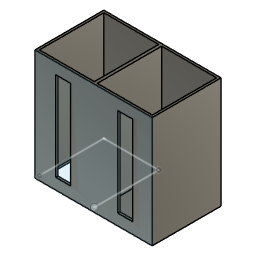
Container (Autodesk Fusion 360 design; units mm, degrees)
Autodesk Fusion 360 part; units mm, degrees
sketch "Szkic1" plane through (0, 0, 0) normal (0, 0, 1) x (1, 0, 0)
  line L0 (0, 0) -> (158.35, 0)
  line L1 (158.35, 0) -> (158.35, 93)
  line L2 (158.35, 93) -> (0, 93)
  line L3 (0, 93) -> (0, 0)
  line L4 (3, 5) -> (3, 3)
  line L5 (3, 3) -> (5, 3)
  line L6 (3, 3) -> (155.35, 3)
  line L7 (155.35, 3) -> (155.35, 90)
  line L8 (155.35, 90) -> (3, 90)
  line L9 (3, 90) -> (3, 3)
  dimension "d1" = 158.35
  dimension "d2" = 93
  dimension "d3" = 152.35
  dimension "d4" = 87
  constraint horizontal L0
  constraint vertical L1
  constraint horizontal L2
  constraint vertical L3
  constraint coincident L0.start L3.end
  constraint horizontal L6
  constraint vertical L7
  constraint horizontal L8
  constraint vertical L9
  measures "d1" distance of L0.start L0.end
  measures "d2" distance of L0.start L2.end
  measures "d3" distance of L4.end L6.end
  measures "d4" distance of L4.end L8.end
extrude "Wyciągnięcie proste1" add sketch "Szkic1" along normal blind 150
sketch "Szkic2" plane through (0, 90, 0) normal (0, -1, 0) x (1, 0, 0)
  line L0 (3, 0) -> (155.35, 0)
  line L1 (155.35, 0) -> (155.35, 150)
  line L2 (155.35, 150) -> (3, 150)
  line L3 (3, 150) -> (3, 0)
  line L4 (79.175, 150) -> (77.175, 150)
  line L5 (77.175, 150) -> (81.175, 150)
  line L6 (81.175, 150) -> (81.175, 0)
  line L7 (81.175, 0) -> (77.175, 0)
  line L8 (77.175, 0) -> (77.175, 150)
  dimension "d7" = 2
  dimension "d8" = 4
  constraint midpoint L2 L4.start
  constraint horizontal L5
  constraint vertical L6
  constraint horizontal L7
  constraint vertical L8
  measures "d7" distance of L4.start L4.end
  measures "d8" distance of L4.end L5.end
extrude "Wyciągnięcie proste2" add sketch "Szkic2" along normal blind 87 contours L0 L2 L4 L5 L6 L7 L8
sketch "Szkic3" plane through (0, 0, 0) normal (0, -1, 0) x (1, 0, 0)
  line L0 (0, 0) -> (158.35, 0)
  line L1 (158.35, 0) -> (158.35, 150)
  line L2 (158.35, 150) -> (0, 150)
  line L3 (0, 150) -> (0, 0)
sketch "Szkic4" plane through (0, 0, 0) normal (0, 0, -1) x (1, 0, 0)
  line L0 (81.175, -3) -> (155.35, -3)
  line L1 (155.35, -3) -> (155.35, -90)
  line L2 (155.35, -90) -> (81.175, -90)
  line L3 (81.175, -90) -> (81.175, -3)
  line L4 (77.175, -3) -> (77.175, -90)
  line L5 (77.175, -90) -> (3, -90)
  line L6 (3, -90) -> (3, -3)
  line L7 (3, -3) -> (77.175, -3)
  line L8 (0, 0) -> (0, -93)
  line L9 (0, -93) -> (158.35, -93)
  line L10 (158.35, -93) -> (158.35, 0)
  line L11 (158.35, 0) -> (0, 0)
  line L12 (0, 0) -> (158.35, 0)
  line L13 (158.35, 0) -> (158.35, -93)
  line L14 (158.35, -93) -> (0, -93)
  line L15 (0, -93) -> (0, 0)
  constraint horizontal L12
  constraint vertical L13
  constraint horizontal L14
  constraint vertical L15
  constraint coincident L9.end L10.start
  constraint coincident L8.start L11.end
extrude "Wyciągnięcie proste3" add sketch "Szkic4" against normal blind 3 contours L0 L1 L2 L3 | L4 L5 L6 L7
sketch "Szkic5" plane through (0, 0, 0) normal (0, -1, 0) x (1, 0, 0)
  line L0 (40, 15) -> (38.0507, 15)
  line L1 (38.0507, 15) -> (28.0507, 15)
  line L2 (28.0507, 15) -> (48.0507, 15)
  line L3 (48.0507, 15) -> (48.0507, 135)
  line L4 (48.0507, 135) -> (28.0507, 135)
  line L5 (28.0507, 135) -> (28.0507, 15)
  line L6 (131.9493, 135) -> (131.9493, 15)
  line L7 (120, 15) -> (121.9493, 15)
  line L8 (111.9493, 135) -> (131.9493, 135)
  line L9 (121.9493, 15) -> (131.9493, 15)
  line L10 (131.9493, 15) -> (111.9493, 15)
  line L11 (111.9493, 15) -> (111.9493, 135)
  dimension "d13" = 10
  dimension "d14" = 20
  dimension "d15" = 120
  constraint horizontal L2
  constraint vertical L3
  constraint horizontal L4
  constraint vertical L5
  measures "d13" distance of L0.end L1.end
  measures "d14" distance of L1.end L2.end
  measures "d15" distance of L1.end L4.end
extrude "Wyciągnięcie proste4" cut sketch "Szkic5" against normal blind 10
sketch "Szkic6" plane through (0, 0, 3) normal (0, 0, 1) x (-1, 0, 0)
  line L0 (-3, -90) -> (-3, -3)
  line L1 (-3, -3) -> (-77.175, -3)
  line L2 (-77.175, -3) -> (-77.175, -90)
  line L3 (-77.175, -90) -> (-3, -90)
  line L4 (-77.175, -3) -> (-77.175, -90)
  line L5 (-77.175, -90) -> (-3, -90)
  line L6 (-3, -90) -> (-3, -3)
  line L7 (-3, -90) -> (-5, -90)
  constraint vertical L4
  constraint horizontal L5
  constraint vertical L6
  constraint coincident L2.end L3.start
  constraint coincident L0.end L1.start
  constraint coincident L5 L7.end
  constraint perpendicular L0 L7
sketch "Szkic7" plane through (0, 0, 3) normal (0, 0, 1) x (-1, 0, 0)
  line L0 (-77.175, -90) -> (-77.175, -3)
  line L1 (-77.175, -3) -> (-77.175, -5)
  line L2 (-75.175, -5) -> (-5, -5)
  line L3 (-5, -5) -> (-5, -88)
  line L4 (-5, -88) -> (-75.175, -88)
  line L5 (-75.175, -88) -> (-75.175, -5)
  point P0 (-5, -90)
  point P1 (-77.175, -3)
  dimension "d18" = 2
  constraint coincident P1 L0.end
  constraint coincident L0 L1.end
  constraint horizontal L2
  constraint vertical L3
  constraint horizontal L4
  constraint vertical L5
  measures "d18" distance of L1.end L2.start
extrude "Wyciągnięcie proste5" cut sketch "Szkic7" against normal blind 10
